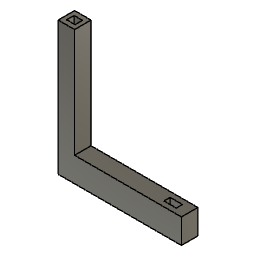
Bras moteur boule v5 (Autodesk Fusion 360 design; units mm, degrees)
Autodesk Fusion 360 part; units mm, degrees
sketch "Esquisse1" plane through (0, 0, 0) normal (0, 0, 1) x (1, 0, 0)
  line L0 (0, 0) -> (8, 0)
  line L1 (8, 0) -> (8, 8)
  line L2 (8, 8) -> (0, 8)
  line L3 (0, 8) -> (0, 0)
  dimension "d1" = 8
  dimension "d2" = 8
  constraint horizontal L0
  constraint vertical L1
  constraint horizontal L2
  constraint vertical L3
  constraint coincident L0.start L3.end
  measures "d1" distance of L1.end L2.end
  measures "d2" distance of L0.start L2.end
extrude "Extrusion1" add sketch "Esquisse1" along normal blind 65
sketch "Esquisse8" plane through (0, 0, 65) normal (0, 0, 1) x (-1, 0, 0)
  line L0 (0, -8) -> (0, 0)
  line L1 (0, 0) -> (-8, 0)
  line L2 (-8, 0) -> (-8, -8)
  line L3 (-8, -8) -> (0, -8)
  line L4 (0, -4) -> (-8, -4)
  line L5 (-1.95, -4) -> (-6.05, -4)
  line L6 (-6.05, -4) -> (-6.05, -5.8)
  line L7 (-6.05, -5.8) -> (-1.95, -5.8)
  line L8 (-1.95, -5.8) -> (-1.95, -4)
  line L9 (-4, -8) -> (-4, 0)
  line L10 (-1.95, -2.2) -> (-1.95, -4)
  line L11 (-6.05, -2.2) -> (-1.95, -2.2)
  line L12 (-6.05, -4) -> (-6.05, -2.2)
  dimension "d41" = 4.1
  dimension "d42" = 2.05
  dimension "d43" = 1.8
  constraint midpoint L0 L4.start
  constraint midpoint L2 L4.end
  constraint horizontal L5
  constraint vertical L6
  constraint horizontal L7
  constraint vertical L8
  constraint coincident L4 L5.start
  constraint midpoint L3 L9.start
  constraint midpoint L1 L9.end
  constraint symmetric L8.end L5 L10.end
  constraint symmetric L6.start L5 L12.start
  constraint symmetric L6.end L5 L11.start
  constraint symmetric L7.end L5 L10.start
  measures "d41" distance of L6 L8
  measures "d42" distance of L8 L9
  measures "d43" distance of L5.start L7.end
extrude "Extrusion8" cut sketch "Esquisse8" against normal blind 6 contours L4 L5 L7 L8 L9 | L4 L5 L9 L10 L11 | L4 L5 L6 L7 L9 | L4 L5 L9 L11 L12
sketch "Esquisse9" plane through (8, 0, 0) normal (1, 0, 0) x (0, 1, 0)
  line L0 (0, 0) -> (8, 0)
  line L1 (8, 0) -> (8, 65)
  line L2 (8, 65) -> (0, 65)
  line L3 (0, 65) -> (0, 0)
  line L4 (0, 0) -> (8, 0)
  line L5 (8, 0) -> (8, 12)
  line L6 (8, 12) -> (0, 12)
  line L7 (0, 12) -> (0, 0)
  dimension "d46" = 12
  constraint horizontal L4
  constraint vertical L5
  constraint horizontal L6
  constraint vertical L7
  constraint coincident L1 L5.end
  constraint coincident L0.start L3.end
  measures "d46" distance of L4 L6
extrude "Extrusion9" add sketch "Esquisse9" along normal blind 52 contours L0 L1 L3 L4 L5 L6 L7
sketch "Esquisse10" plane through (0, 0, 12) normal (0, 0, 1) x (-1, 0, 0)
  line L0 (-8, -8) -> (-8, 0)
  line L1 (-8, 0) -> (-60, 0)
  line L2 (-60, 0) -> (-60, -8)
  line L3 (-60, -8) -> (-8, -8)
  line L4 (-55, -5.5) -> (-49, -5.5)
  line L5 (-49, -5.5) -> (-49, -2.5)
  line L6 (-49, -2.5) -> (-55, -2.5)
  line L7 (-55, -2.5) -> (-55, -5.5)
  dimension "d49" = 2.5
  dimension "d50" = 2.5
  dimension "d51" = 5
  dimension "d52" = 6
  constraint horizontal L4
  constraint vertical L5
  constraint horizontal L6
  constraint vertical L7
  measures "d49" distance of L3 L4
  measures "d50" distance of L1 L6
  measures "d51" distance of L2 L7
  measures "d52" distance of L5 L7
extrude "Extrusion10" cut sketch "Esquisse10" against normal blind 23 contours L4 L5 L6 L7
